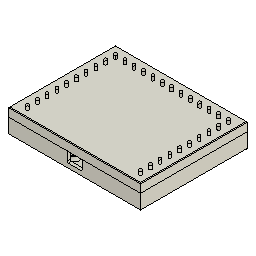
AZ-Oneboard Gehäuse (Autodesk Fusion 360 design; units mm, degrees)
Autodesk Fusion 360 part; units mm, degrees
note: some values were not read from the file. Set by a fixed rule: which sketch regions a step uses.
sketch "Skizze1" plane through (0, 0, 0) normal (0, 0, 1) x (1, 0, 0)
  line L0 (23.9395, -25.3365) -> (-23.9395, -25.3365) construction
  line L1 (-23.9395, -25.3365) -> (-23.9395, 25.3365) construction
  line L2 (-23.9395, 25.3365) -> (23.9395, 25.3365) construction
  line L3 (23.9395, 25.3365) -> (23.9395, -25.3365) construction
  line L4 (23.9395, -25.3365) -> (-23.9395, 25.3365) construction
  line L5 (-23.9395, -25.3365) -> (23.9395, 25.3365) construction
  dimension "d4" = 47.879
  dimension "d5" = 50.673
  constraint horizontal L0
  constraint perpendicular L0 L1
  constraint parallel L0 L2
  constraint parallel L1 L3
  constraint coincident L4 origin
  constraint coincident L5 origin
  measures "d4" distance of L1.end L2.end
  measures "d5" distance of L0.end L1.end
sketch "Skizze5" plane through (0, 0, 0) normal (0, 0, 1) x (1, 0, 0) in component "UnteresGehauese"
  line L0 (0, 59) -> (0, -37)
  line L1 (-17.5898, 22.5898) -> (16.4102, 22.5898)
  line L2 (-20, -21.701) -> (22, -21.701)
  line L3 (-8.8265, 28) -> (-8.8265, -29)
  line L4 (8.8265, 28) -> (8.8265, -27)
  circle A0 centre (-8.8265, 22.5898) radius 2.5
  circle A1 centre (8.8265, 22.5898) radius 2.5
  circle A2 centre (-8.8265, 22.5898) radius 1.175
  circle A3 centre (8.8265, 22.5898) radius 1.175
  circle A4 centre (-8.8265, -21.701) radius 2.5
  circle A5 centre (8.8265, -21.701) radius 2.5
  circle A6 centre (-8.8265, -21.701) radius 1.175
  circle A7 centre (8.8265, -21.701) radius 1.175
  line L5 (-52.5, 55) -> (52.5, 55)
  line L6 (52.5, 55) -> (52.5, -30)
  line L7 (52.5, -30) -> (-52.5, -30)
  line L8 (-52.5, -30) -> (-52.5, 55)
  line L9 (51, -28.5) -> (-51, -28.5)
  line L10 (-51, -28.5) -> (-51, 53.5)
  line L11 (-51, 53.5) -> (51, 53.5)
  line L12 (51, 53.5) -> (51, -28.5)
  line L13 (50, -27.5) -> (-50, -27.5)
  line L14 (-50, -27.5) -> (-50, 52.5)
  line L15 (-50, 52.5) -> (50, 52.5)
  line L16 (50, 52.5) -> (50, -27.5)
  line L17 (-67, 32.5) -> (64, 32.5) construction
  line L18 (-35, 59) -> (-35, 25) construction
  line L19 (35, 59) -> (35, 26) construction
  circle A8 centre (-35, 32.5) radius 2.5
  circle A9 centre (-35, 22.5) radius 5
  line L20 (-37.5, 32.5) -> (-37.5, 28)
  line L21 (-32.5, 32.5) -> (-32.5, 28)
  arc A10 (-38.2877, 26.2671) -> (-37.5, 28) centre (-39.8, 28) ccw
  arc A11 (-32.5, 28) -> (-31.7123, 26.2671) centre (-30.2, 28) ccw
  line L22 (-39.8366, 28) -> (-31.3098, 28) construction
  circle A12 centre (35, 32.5) radius 2.5
  line L23 (37.5, 32.5) -> (37.5, 28)
  line L24 (32.5, 32.5) -> (32.5, 28)
  arc A13 (31.7123, 26.2671) -> (32.5, 28) centre (30.2, 28) ccw
  circle A14 centre (35, 22.5) radius 5
  arc A15 (37.5, 28) -> (38.2877, 26.2671) centre (39.8, 28) ccw
  dimension "d6" = 17.653
  dimension "d7" = 2.35
  dimension "d8" = 2.35
  dimension "d9" = 5
  dimension "d10" = 5
  dimension "d11" = 5
  dimension "d12" = 5
  dimension "d13" = 2.35
  dimension "d14" = 2.35
  dimension "d15" = 105
  dimension "d16" = 55
  dimension "d17" = 30
  dimension "d18" = 1.5
  dimension "d19" = 2.5
  dimension "d77" = 20
  dimension "d78" = 70
  dimension "d79" = 5
  dimension "d81" = 10
  dimension "d83" = 10
  dimension "d85" = 4.5
  dimension "d86" = 2.3
  dimension "d87" = 2.3
  constraint vertical L0
  constraint perpendicular L0 L1
  constraint perpendicular L0 L2
  constraint coincident L0 origin
  constraint perpendicular L1 L3
  constraint perpendicular L1 L4
  constraint coincident L3 A0.centre
  constraint coincident L1 A0.centre
  constraint coincident L1 A1.centre
  constraint coincident L4 A1.centre
  constraint concentric A0 A2
  constraint concentric A1 A3
  constraint coincident L2 A4.centre
  constraint coincident L3 A4.centre
  constraint coincident L2 A5.centre
  constraint coincident L4 A5.centre
  constraint concentric A4 A6
  constraint concentric A5 A7
  constraint horizontal L5
  constraint vertical L6
  constraint horizontal L7
  constraint vertical L8
  constraint symmetric L0 L6 L8
  constraint perpendicular L6 L17
  constraint perpendicular L15 L18
  constraint perpendicular L17 L19
  constraint coincident L17 A8.centre
  constraint coincident L18 A8.centre
  constraint coincident L18 A9.centre
  constraint coincident A8 L20.start
  constraint coincident L17 L20.start
  constraint tangent A8 L20
  constraint coincident A8 L21.start
  constraint coincident L17 L21.start
  constraint tangent A8 L21
  constraint coincident A9 A10.start
  constraint tangent L20 A10
  constraint coincident A9 A11.end
  constraint tangent L21 A11
  constraint perpendicular L21 L22
  constraint coincident L20.end L22
  constraint coincident L21.end L22
  constraint symmetric L0 A8 A12
  constraint symmetric L0 A9 A14
  constraint symmetric L0 L20.start L23.start
  constraint symmetric L0 L20.end L23.end
  constraint symmetric L0 L21.start L24.start
  constraint symmetric L0 L21.end L24.end
  constraint symmetric L0 A10.start A15.end
  constraint symmetric L0 A10 A15
  constraint symmetric L0 A11.end A13.start
  constraint symmetric L0 A11 A13
  measures "d7" diameter of A2
  measures "d8" diameter of A3
  measures "d9" diameter of A0
  measures "d10" diameter of A1
  measures "d11" diameter of A4
  measures "d12" diameter of A5
  measures "d13" diameter of A6
  measures "d14" diameter of A7
  measures "d16" distance of L5 origin
  measures "d17" distance of origin L7
  measures "d77" distance of L15 L17
  measures "d78" distance of L18 L19
  measures "d79" diameter of A8
  measures "d81" diameter of A9
  measures "d83" distance of A8.centre A9.centre
  measures "d85" distance of A8.centre L22
  measures "d86" radius of A10
  measures "d87" radius of A11
extrude "Extrusion1" add sketch "Skizze5" against normal blind 2 contours L0 L5 L6 L7 L9 L11 L12 | L0 L5 L7 L8 L9 L10 L11 | L0 L9 L11 L12 L13 L15 L16 | L0 L3 L9 L10 L11 L13 L14 L15 | L0 L1 L2 L4 A1 A5 L13 L15 L16 | L0 L1 L3 A0 A4 L13 L14 L15 | L0 L1 L2 L4 A1 A5 | L0 L1 L2 L3 A0 A4 | L0 L2 L3 A4 L13 | L1 L3 A0 A2 | L1 L3 A0 A2 | L1 L4 A1 A3 | L1 L4 A1 A3 | L0 L3 L9 L13 | L2 L3 A4 A6 | L2 L3 A4 A6 | L2 L4 A5 A7 | L2 L4 A5 A7 | L1 L3 A2 | L1 L3 A2 | L1 L3 A0 A2 | L1 L3 A0 A2 | L1 L4 A3 | L1 L4 A3 | L1 L4 A1 A3 | L1 L4 A1 A3 | L2 L3 A6 | L2 L3 A6 | L2 L3 A4 A6 | L2 L3 A4 A6 | L2 L4 A7 | L2 L4 A7 | L2 L4 A5 A7 | L2 L4 A5 A7 | L1 L3 A2 | L1 L3 A2 | L1 L4 A3 | L1 L4 A3 | L2 L3 A6 | L2 L3 A6 | L2 L4 A7 | L2 L4 A7 | A8 | A8 A9 L20 L21 A10 A11 | A9 | A12 | A12 L23 L24 A13 A14 A15 | A14 makes body 1 in component "UnteresGehauese"
extrude "Extrusion2" add sketch "Skizze5" along normal blind 10 contours L0 L5 L6 L7 L9 L11 L12 | L0 L5 L7 L8 L9 L10 L11 bodies 1 in component "UnteresGehauese"
extrude "Extrusion3" add sketch "Skizze5" along normal blind 13 contours L0 L9 L11 L12 L13 L15 L16 | L0 L3 L9 L10 L11 L13 L14 L15 | L0 L3 L9 L13 bodies 1 in component "UnteresGehauese"
extrude "Extrusion4" add sketch "Skizze5" along normal blind 3 contours L1 L3 A0 A2 | L1 L3 A0 A2 | L1 L4 A1 A3 | L1 L4 A1 A3 | L2 L3 A4 A6 | L2 L3 A4 A6 | L2 L4 A5 A7 | L2 L4 A5 A7 | L1 L3 A0 A2 | L1 L3 A0 A2 | L1 L4 A1 A3 | L1 L4 A1 A3 | L2 L3 A4 A6 | L2 L3 A4 A6 | L2 L4 A5 A7 | L2 L4 A5 A7 bodies 1 in component "UnteresGehauese"
fillet "Abrundung2" radius 2 4 edges at (-11.1573, -20.7969, 0) (6.4957, -20.7969, 0) (-11.1573, 23.4938, 0) (6.4957, 23.4938, 0) on bodies 1 in component "UnteresGehauese"
sketch "Skizze6" plane through (0, -30, 0) normal (0, -1, 0) x (1, 0, 0) in component "UnteresGehauese"
  line L0 (-52.5, 10) -> (-52.5, -2)
  line L1 (-52.5, -2) -> (52.5, -2)
  line L2 (52.5, -2) -> (52.5, 10)
  line L3 (52.5, 10) -> (-52.5, 10)
  line L4 (6, 13) -> (6, 3)
  line L5 (5, 2) -> (-5, 2)
  line L6 (-6, 3) -> (-6, 13)
  line L7 (52.5, 0) -> (-52.5, 0)
  line L8 (0, 22.606) -> (0, -13)
  arc A0 (5, 2) -> (6, 3) centre (5, 3) ccw
  arc A1 (-6, 3) -> (-5, 2) centre (-5, 3) ccw
  line L9 (-51, 13) -> (51, 13)
  point P0 (6, 9)
  point P1 (6, 2)
  dimension "d32" = 2
  dimension "d34" = 12
  dimension "d35" = 1
  dimension "d48" = 1
  constraint vertical L4
  constraint horizontal L5
  constraint vertical L6
  constraint perpendicular L1 L8
  constraint coincident L8 origin
  constraint symmetric L4 L6 L8
  constraint coincident P1 L4
  constraint coincident P1 L5
  constraint tangent L4 A0
  constraint tangent L5 A0
  constraint coincident P0 L4
  constraint tangent L5 A1
  constraint tangent L6 A1
  constraint coincident L4.start L9
  constraint coincident L6.end L9
  measures "d32" distance of L5 L7
  measures "d34" distance of L4 L6
  measures "d35" radius of A0
  measures "d48" radius of A1
extrude "Extrusion5" cut sketch "Skizze6" against normal up to surface (2.5 mm away) contours L3 L6 L8 L9 | L3 L5 L6 L8 A1 | L3 L4 L8 L9 | L3 L4 L5 L8 A0 bodies 1 in component "UnteresGehauese"
sketch "Skizze1 (2)" plane through (0, 0, 13) normal (0, 0, 1) x (-1, 0, 0) in component "ObereGehauese"
  line L0 (50, -52.5) -> (-50, -52.5)
  line L1 (-50, -52.5) -> (-50, 27.5)
  line L2 (6, 27.5) -> (50, 27.5)
  line L3 (50, 27.5) -> (50, -52.5)
  line L4 (-51, -53.5) -> (51, -53.5)
  line L5 (51, -53.5) -> (51, 28.5)
  line L6 (-6, 28.5) -> (-51, 28.5)
  line L7 (-51, 28.5) -> (-51, -53.5)
  line L8 (52.5, -55) -> (-52.5, -55)
  line L9 (52.5, 30) -> (52.5, -55)
  line L10 (-52.5, 30) -> (52.5, 30)
  line L11 (-52.5, -55) -> (-52.5, 30)
  line L12 (51.05, 28.55) -> (-51.05, 28.55)
  line L13 (-51.05, 28.55) -> (-51.05, -53.55)
  line L14 (-51.05, -53.55) -> (51.05, -53.55)
  line L15 (51.05, -53.55) -> (51.05, 28.55)
  line L16 (6, 28.5) -> (6, 27.5)
  line L17 (-50, 27.5) -> (-6, 27.5)
  line L18 (-6, 27.5) -> (-6, 28.5)
  line L19 (51, 28.5) -> (6, 28.5)
  line L20 (-51, -53.5) -> (-51, 28.5)
extrude "Extrusion2'" add sketch "Skizze1 (2)" along normal up to surface (-3 mm away) and the other way blind -2 separate body contours L8 L9 L10 L11 makes body 2 in component "ObereGehauese"
sketch "Skizze2" plane through (0, 0, 15) normal (0, 0, 1) x (-1, 0, 0) in component "ObereGehauese"
  line L0 (51.05, 28.55) -> (51.05, -53.55)
  line L1 (51.05, -53.55) -> (-51.05, -53.55)
  line L2 (-51.05, -53.55) -> (-51.05, 28.55)
  line L3 (-51.05, 28.55) -> (51.05, 28.55)
  line L4 (-52.5, -55) -> (52.5, -55)
  line L5 (52.5, -55) -> (52.5, 30)
  line L6 (52.5, 30) -> (-52.5, 30)
  line L7 (-52.5, 30) -> (-52.5, -55)
  line L8 (52.5, -55) -> (-52.5, -55)
  line L9 (52.5, 30) -> (52.5, -55)
  line L10 (-52.5, -55) -> (-52.5, 30)
  line L11 (-52.5, 30) -> (52.5, 30)
extrude "Extrusion3'" add sketch "Skizze2" along normal blind 2 contours L0 L1 L2 L3 | L4 L5 L6 L7 L8 L9 L10 L11 bodies 2 in component "ObereGehauese"
fillet "Abrundung3" radius 0.5 5 edges at (-28.5, -28.5, 13) (-51, 12.5, 13) (28.5, -28.5, 13) (51, 12.5, 13) (0, 53.5, 13) on bodies 1 in component "UnteresGehauese"
fillet "Abrundung4" radius 0.5 1 faces at (17.5, -1.6667, -2) on bodies 1 in component "UnteresGehauese"
fillet "Abrundung1" radius 0.5 1 faces at (17.5, -1.6667, 17) on bodies 2 in component "ObereGehauese"
sketch "Skizze3" plane through (0, 0, 17) normal (0, 0, 1) x (-1, 0, 0) in component "ObereGehauese"
  line L0 (52, -54.5) -> (52, 29.5)
  line L1 (52, 29.5) -> (-52, 29.5)
  line L2 (-52, 29.5) -> (-52, -54.5)
  line L3 (-52, -54.5) -> (52, -54.5)
  line L4 (47.7071, -48.7929) -> (44.1716, -45.2574)
  line L5 (46.2929, -50.2071) -> (42.7574, -46.6716)
  line L6 (46.6958, -51.4903) -> (46.6958, -41) construction
  arc A0 (46.2929, -50.2071) -> (47.7071, -48.7929) centre (47, -49.5) ccw
  arc A1 (44.1716, -45.2574) -> (42.7574, -46.6716) centre (43.4645, -45.9645) ccw
  line L7 (47.7071, -48.7929) -> (45.2596, -51.2404) construction
  line L8 (44.1716, -45.2574) -> (42.887, -46.542) construction
  dimension "d56" = 45
  dimension "d57" = 5
  dimension "d58" = 2
  dimension "d59" = 5
  dimension "d60" = 5
  constraint parallel L4 L5
  constraint vertical L6
  constraint tangent L5 A0
  constraint tangent L5 A1
  constraint perpendicular L4 L7
  constraint coincident L5.start L7
  constraint perpendicular L4 L8
  constraint coincident L5.end L8
  measures "d56" angle of L4 L6
  measures "d57" distance of L7 L8
  measures "d58" distance of L4 L5
  measures "d59" distance of L3 A0.centre
  measures "d60" distance of L0 A0.centre
extrude "Extrusion4'" cut sketch "Skizze3" against normal up to surface (2 mm away) contours L4 L5 A0 A1 bodies 2 in component "ObereGehauese"
pattern_linear "R-Anordnung2" count 10 spacing 7.7778 along (0, -1, 0) count 2 spacing 90 along (1, 0, 0) of "Extrusion4'" in component "ObereGehauese"
pattern_linear "R-Anordnung3" count 12 spacing 7.4545 along (1, 0, 0) of "Extrusion4'" in component "ObereGehauese"
extrude "Extrusion6" cut sketch "Skizze5" against normal through all contours L1 L3 A2 | L1 L3 A2 | L1 L4 A3 | L1 L4 A3 | L2 L3 A6 | L2 L3 A6 | L2 L4 A7 | L2 L4 A7 | L1 L3 A2 | L1 L3 A2 | L1 L4 A3 | L1 L4 A3 | L2 L3 A6 | L2 L3 A6 | L2 L4 A7 | L2 L4 A7 bodies 1 in component "UnteresGehauese"
extrude "Extrusion7" cut sketch "Skizze5" against normal through all contours A8 | A8 A9 L20 L21 A10 A11 | A9 | A12 | A12 L23 L24 A13 A14 A15 | A14 bodies 1 in component "UnteresGehauese"
pattern_linear "R-Anordnung1" [suppressed] in component "ObereGehauese"
fillet "Abrundung1'" [suppressed] in component "UnteresGehauese"
component "UnteresGehauese" placed x (1, 0, 0) y (0, 1, 0) z (0, 0, 1) at (0, 0, 0)
component "ObereGehauese" placed x (1, 0, 0) y (0, 1, 0) z (0, 0, 1) at (0, 0, 0)
equation "d7 = InnenDurchmesserBefestigungsloch"
equation "d8 = InnenDurchmesserBefestigungsloch"
equation "d13 = InnenDurchmesserBefestigungsloch"
equation "d14 = InnenDurchmesserBefestigungsloch"
equation "InnenDurchmesserBefestigungsloch = 2.35 mm"
